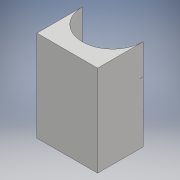
# Autodesk Inventor part: 38
Saved by Autodesk Inventor 2017 (Build 210142000, 142)
## iProperties
Part Number: 38
Material: 一般
Document SubType Name: Modeling
Designer: Brian
Density: 1 g/cm^3
Appearance: 預設
Author: Brian
Autodesk Inventor part; units mm, degrees
ref_plane "YZ Plane" through (0, 0, 0) normal (1, 0, 0) x (0, 1, 0)
ref_plane "XZ Plane" through (0, 0, 0) normal (0, 1, 0) x (-1, 0, 0)
ref_plane "XY Plane" through (0, 0, 0) normal (0, 0, 1) x (1, 0, 0)
sketch "草圖1" plane through (0, 0, 0) normal (0, 1, 0) x (-1, 0, 0)
  line L0 (0, 0) -> (-40, 0)
  line L1 (-40, 0) -> (-40, -60)
  line L2 (-40, -60) -> (0, -60)
  line L3 (0, -60) -> (0, 0)
  dimension "d0" = 40
  dimension "d1" = 60
  constraints: 8 end point, 2 parallel, 1 horizontal, 1 perpendicular
  measures "d0" distance of L1.end L2.end
  measures "d1" distance of L0.end L1.end
extrude "擠出1" add sketch "草圖1" along normal blind 30
sketch "草圖2" plane through (0, 0, 0) normal (0, 0, 1) x (1, 0, 0)
  line L0 (0, 30) -> (40, 30) projected
  circle A0 centre (20, 30) radius 20
  point P0 (0, 0)
  constraints: 1 horizontal alignment, 1 midpoint, 2 other
extrude "擠出2" cut sketch "草圖2" against normal blind 20
sketch "草圖3" plane through (0, 0, -20) normal (0, 0, 1) x (1, 0, 0)
  arc A0 (0, 30) -> (40, 30) centre (20, 30) ccw projected
  line L0 (40, 30) -> (20, 10)
  line L1 (40, 30) -> (0, 30) projected
  line L2 (20, 10) -> (0, 30)
  line L3 (0, 30) -> (40, 30)
  point P0 (0, 0)
  constraints: 6 end point, 1 collinear, 1 perpendicular, 1 point on circle
extrude "擠出3" cut sketch "草圖3" against normal blind 20 contours L1 L0 L2
